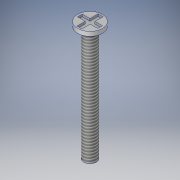
# Autodesk Inventor part: srew long
Saved by Autodesk Inventor 2018 (Build 220112000, 112)
## iProperties
Created: 2018-03-02
Part Number: srew long
Material: Aluminum 6061
Document SubType Name: Modeling
Designer: 238438
Density: 2.7 g/cm^3
Appearance: Aluminum - Flat
Mass: 0.12708 g
Surface Area: 1.23988 cm^2
Volume: 0.0470666 cm^3
Author: 238438
Autodesk Inventor part; units mm, degrees
ref_plane "YZ Plane" through (0, 0, 0) normal (1, 0, 0) x (0, 1, 0)
ref_plane "XZ Plane" through (0, 0, 0) normal (0, 1, 0) x (-1, 0, 0)
ref_plane "XY Plane" through (0, 0, 0) normal (0, 0, 1) x (1, 0, 0)
sketch "Sketch1" plane through (0, 0, 0) normal (0, 0, 1) x (1, 0, 0)
  line L0 (0, 0) -> (1.778, 0)
  line L1 (1.778, 0) -> (1.778, -0.6096)
  line L2 (1.778, -0.6096) -> (0.9017, -0.6096)
  line L3 (0.9017, -0.6096) -> (0.9017, -17.1196)
  line L4 (0.9017, -17.1196) -> (0, -17.1196)
  line L5 (0, -17.1196) -> (0, 0)
  line L6 (0, 0) -> (0, -18.8505)
  dimension "d0" = 1.778
  dimension "d1" = 0.6096
  dimension "d2" = 0.8763
  dimension "d3" = 16.51
  dimension "d5" = 90
  dimension "d6" = 90
  constraints: 14 end point, 4 perpendicular, 1 horizontal, 1 vertical
  measures "d0" distance of L0.start L0.end
  measures "d1" distance of L0.end L1.end
  measures "d2" distance of L1.end L2.end
  measures "d3" distance of L2.end L3.end
  measures "d5" angle of L3 L4
  measures "d6" angle of L5 L4
revolve "Revolution1" add sketch "Sketch1" angle 360 about axis through (0, 0, 0) along (0, -1, 0)
thread "Thread1" size "1-64 UNC" class "2A" standard "ANSI Unified Screw Threads" full length
sketch "Sketch2" plane through (0, 0, 0) normal (0, 1, 0) x (1, 0, 0)
  line L0 (-1.4599, 0.343) -> (-1.4599, -0.3293)
  line L1 (1.4436, -0.3293) -> (1.4436, 0.343)
  line L2 (-0.3517, -1.5261) -> (0.3649, -1.5261)
  line L3 (0.3649, 1.5177) -> (-0.3517, 1.5177)
  line L4 (0.3649, -1.5261) -> (0.3649, -0.3293)
  line L5 (0.3649, 0.343) -> (0.3649, 1.5177)
  line L6 (1.4436, 0.343) -> (0.3649, 0.343)
  line L7 (-0.3517, 0.343) -> (-1.4599, 0.343)
  line L8 (-1.4599, -0.3293) -> (-0.3517, -0.3293)
  line L9 (0.3649, -0.3293) -> (1.4436, -0.3293)
  line L10 (-0.3517, 1.5177) -> (-0.3517, 0.343)
  line L11 (-0.3517, -0.3293) -> (-0.3517, -1.5261)
  point P0 (0, 0)
  constraints: 24 end point, 10 parallel, 4 perpendicular, 3 horizontal
extrude "Extrusion1" cut sketch "Sketch2" against normal blind 0.3175
body "Solid1"
